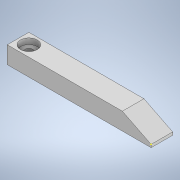
# Autodesk Inventor part: cuña 10cm
Saved by Autodesk Inventor 2021 (Build 250183000, 183)
## iProperties
Created: 2022-09-17
Part Number: cuña 10cm
Material: Genérico
Document SubType Name: Modeling
Designer: sergi
Density: 1 g/cm^3
Appearance: Valor por defecto
Author: sergi
Autodesk Inventor part; units mm, degrees
ref_plane "YZ Plane" through (0, 0, 0) normal (1, 0, 0) x (0, 1, 0)
ref_plane "XZ Plane" through (0, 0, 0) normal (0, 1, 0) x (-1, 0, 0)
ref_plane "XY Plane" through (0, 0, 0) normal (0, 0, 1) x (1, 0, 0)
sketch "Boceto1" plane through (0, 0, 0) normal (0, 1, 0) x (-1, 0, 0)
  line L0 (0, 0) -> (100, 0)
  line L1 (100, 0) -> (100, -15)
  line L2 (100, -15) -> (0, -15)
  line L3 (0, -15) -> (0, 0)
  dimension "d0" = 100
  dimension "d1" = 15
  constraints: 8 end point, 2 parallel, 1 horizontal, 1 perpendicular
  measures "d0" distance of L1.end L2.end
  measures "d1" distance of L0.end L1.end
extrude "Extrusión1" add sketch "Boceto1" along normal blind 10
sketch "Boceto3" plane through (0, 0, 0) normal (1, 0, 0) x (0, 0, -1)
  point P0 (0, 0)
chamfer "Chaflán1" distance 20 distance2 10 1 edges at (0, 10, -7.5) measured on face at (-33.3333, 10, -5)
sketch "Boceto4" plane through (0, 0, 0) normal (0, -1, 0) x (1, 0, 0)
  line L0 (0, -15) -> (-100, -15) projected
  line L1 (0, -15) -> (-100, -15)
  line L2 (-100, -15) -> (-100, 0)
  line L3 (-100, 0) -> (0, 0)
  line L4 (0, 0) -> (0, -15)
  dimension "d25" = 100
  constraints: 8 end point, 2 parallel, 1 horizontal, 1 perpendicular
  measures "d25" distance of L2.end L3.end
extrude "Extrusión2" add sketch "Boceto4" along normal blind 2
sketch "Boceto6" plane through (0, 10, 0) normal (0, 1, 0) x (1, 0, 0)
  line L0 (-100, 15) -> (-100, 0) projected
  line L1 (-100, 0) -> (-20, 0) projected
  point P0 (0, 0)
  point P1 (-92.5, 7.5)
  dimension "d26" = 7.5
  dimension "d27" = 7.5
  measures "d26" distance from line of L0 point (-92.5, 7.5)
  measures "d27" distance from line of L1 point (-92.5, 7.5)
hole "Agujero3" at (-92.5, 10, -7.5) direction (0, -1, 0) diameter 5.2 end through all counterbore diameter 11.7 counterbore depth 4
